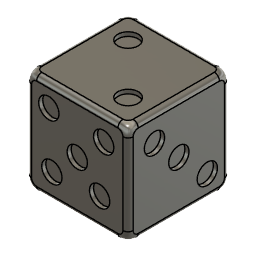
Dice (Autodesk Fusion 360 design; units mm, degrees)
part number: 2026-05-17-14-31-05-637
Autodesk Fusion 360 part; units mm, degrees
box "BoxPrimitive2" add length 50 width 50 height 50 placed x (0, 0, -1) y (-1, 0, 0) z (0, 1, 0) at (50, 0, 0)
sketch "Sketch8" plane through (0, 0, 0) normal (0, 1, 0) x (1, 0, 0)
  circle A0 centre (25, 25) radius 5
  dimension "diahole" = 10
  measures "diahole" diameter of A0
extrude "Extrude3" cut sketch "Sketch8" along normal blind 2
sketch "Sketch9" plane through (0, 50, 0) normal (0, 1, 0) x (-1, 0, 0)
  line L0 (-50, -50) -> (0, -50)
  line L1 (0, -50) -> (0, 0)
  line L2 (0, 0) -> (-50, 0)
  line L3 (-50, 0) -> (-50, -50)
  circle A0 centre (-12.5, -37.5) radius 5
  circle A1 centre (-37, -13) radius 5
  dimension "d75" = 10
  dimension "d76" = 10
  measures "d75" diameter of A0
  measures "d76" diameter of A1
extrude "Extrude4" cut sketch "Sketch9" against normal blind 2 contours A0 | A1
sketch "Sketch10" plane through (50, 0, 0) normal (1, 0, 0) x (0, 0, -1)
  line L0 (0, 50) -> (0, 0)
  line L1 (0, 0) -> (50, 0)
  line L2 (50, 0) -> (50, 50)
  line L3 (50, 50) -> (0, 50)
  circle A0 centre (39, 11) radius 5
  circle A1 centre (25, 25) radius 5
  circle A2 centre (13, 37) radius 5
  dimension "d79" = 10
  dimension "d80" = 10
  measures "d79" diameter of A0
  measures "d80" diameter of A1
extrude "Extrude5" cut sketch "Sketch10" against normal blind 2 contours A0 | A1 | A2
sketch "Sketch11" plane through (0, 0, 0) normal (0, 0, 1) x (1, 0, 0)
  line L0 (0, 50) -> (0, 0)
  line L1 (0, 0) -> (50, 0)
  line L2 (50, 0) -> (50, 50)
  line L3 (50, 50) -> (0, 50)
  circle A0 centre (25, 25) radius 5
  circle A1 centre (11, 39) radius 5
  circle A2 centre (12.5, 12.5) radius 5
  circle A3 centre (38, 38) radius 5
  circle A4 centre (36, 14) radius 5
  dimension "d83" = 10
  dimension "d84" = 10
  dimension "d85" = 10
  dimension "d86" = 10
  dimension "d87" = 10
  measures "d83" diameter of A0
  measures "d84" diameter of A1
  measures "d85" diameter of A2
  measures "d86" diameter of A3
  measures "d87" diameter of A4
extrude "Extrude6" cut sketch "Sketch11" against normal blind 2 contours A0 | A1 | A2 | A3 | A4
sketch "Sketch12" plane through (0, 0, -50) normal (0, 0, -1) x (-1, 0, 0)
  line L0 (-50, 50) -> (-50, 0)
  line L1 (-50, 0) -> (0, 0)
  line L2 (0, 0) -> (0, 50)
  line L3 (0, 50) -> (-50, 50)
  circle A0 centre (-39, 39) radius 5
  circle A1 centre (-37.5, 12.5) radius 5
  circle A2 centre (-12.5, 38.594) radius 5
  circle A3 centre (-14, 14) radius 5
  dimension "d90" = 10
  dimension "d91" = 10
  dimension "d92" = 10
  dimension "d93" = 10
  measures "d90" diameter of A0
  measures "d91" diameter of A1
  measures "d92" diameter of A2
  measures "d93" diameter of A3
extrude "Extrude7" cut sketch "Sketch12" against normal blind 2 contours A0 | A1 | A2 | A3
sketch "Sketch13" plane through (0, 0, 0) normal (-1, 0, 0) x (0, 0, 1)
  line L0 (-50, 50) -> (-50, 0)
  line L1 (-50, 0) -> (0, 0)
  line L2 (0, 0) -> (0, 50)
  line L3 (0, 50) -> (-50, 50)
  circle A0 centre (-39, 39) radius 5
  circle A1 centre (-39, 25) radius 5
  circle A2 centre (-39, 11) radius 5
  circle A3 centre (-13, 25) radius 5
  circle A4 centre (-12.5, 37.5) radius 5
  circle A5 centre (-12.5, 12.5) radius 5
  dimension "d96" = 10
  dimension "d97" = 10
  dimension "d99" = 10
  dimension "d100" = 10
  dimension "d101" = 10
  dimension "d102" = 10
  measures "d96" diameter of A0
  measures "d97" diameter of A1
  measures "d99" diameter of A2
  measures "d100" diameter of A3
  measures "d101" diameter of A4
  measures "d102" diameter of A5
extrude "Extrude8" cut sketch "Sketch13" against normal blind 2 contours A0 | A1 | A2 | A3 | A4 | A5
fillet "Fillet1" radius 2.5 12 edges at (25, 50, 0) (50, 50, -25) (25, 50, -50) (0, 50, -25) (0, 25, -50) (0, 25, 0) (50, 25, 0) (50, 25, -50) (50, 0, -25) (25, 0, 0) (0, 0, -25) (25, 0, -50)
